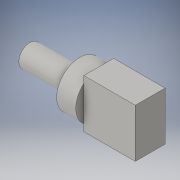
# Autodesk Inventor part: Switch
Saved by Autodesk Inventor 2016 (Build 200138000, 138)
## iProperties
Created: 2017-09-11
Part Number: Switch
Material: Generic
Document SubType Name: Modeling
Designer: student
Density: 1 g/cm^3
Appearance: Default
Author: student
Autodesk Inventor part; units mm, degrees
ref_plane "YZ Plane" through (0, 0, 0) normal (1, 0, 0) x (0, 1, 0)
ref_plane "XZ Plane" through (0, 0, 0) normal (0, 1, 0) x (-1, 0, 0)
ref_plane "XY Plane" through (0, 0, 0) normal (0, 0, 1) x (1, 0, 0)
sketch "Sketch1" plane through (0, 0, 0) normal (0, 0, 1) x (1, 0, 0)
  line L0 (0, 0) -> (-13.6398, 0)
  line L1 (-13.6398, 0) -> (-13.6398, -12.9032)
  line L2 (-13.6398, -12.9032) -> (0, -12.9032)
  line L3 (0, -12.9032) -> (0, 0)
  dimension "d0" = 13.6398
  dimension "d1" = 12.9032
  constraints: 8 end point, 2 parallel, 1 horizontal, 1 perpendicular
  measures "d0" distance of L2.end L1.end
  measures "d1" distance of L2.end L0.start
extrude "Extrusion1" add sketch "Sketch1" along normal blind 7.8994
sketch "Sketch2" plane through (-13.6398, -12.9032, 0) normal (-1, 0, 0) x (0, 0, 1)
  circle A0 centre (3.9497, 6.4516) radius 6.096
  point P0 (0, 12.9032)
  dimension "d4" = 12.192
  constraints: 1 centre point
  measures "d4" diameter of A0
extrude "Extrusion2" add sketch "Sketch2" along normal blind 5.08
sketch "Sketch3" plane through (-18.7198, -6.4516, 3.9497) normal (-1, 0, 0) x (0, 0, 1)
  circle A0 centre (0, 0) radius 2.921
  point P0 (-3.9497, 6.4516)
  dimension "d7" = 5.842
  constraints: 1 centre point
  measures "d7" diameter of A0
extrude "Extrusion3" add sketch "Sketch3" along normal blind 13.208
body "Solid1"
